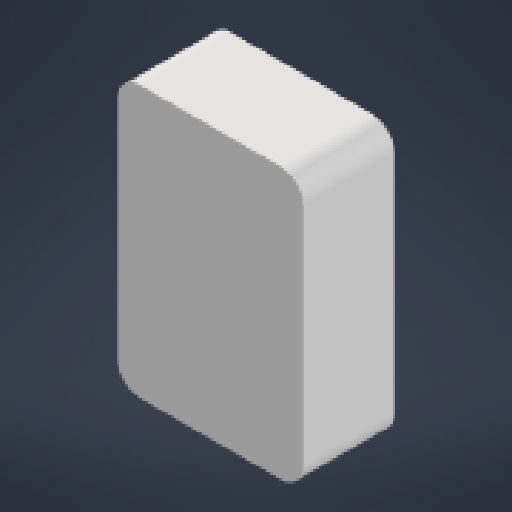
# Autodesk Inventor part: RPI
Saved by Autodesk Inventor 2026.1 (Build 301233020, 233B)
## iProperties
Created: 2025-10-22
Part Number: RPI
Material: Generic
Document SubType Name: Modeling
Designer: Malthe Sennels
Density: 1 g/cm^3
Appearance: Default
Author: Malthe Sennels
Autodesk Inventor part; units mm, degrees
ref_plane "YZ Plane" through (0, 0, 0) normal (1, 0, 0) x (0, 1, 0)
ref_plane "XZ Plane" through (0, 0, 0) normal (0, 1, 0) x (-1, 0, 0)
ref_plane "XY Plane" through (0, 0, 0) normal (0, 0, 1) x (1, 0, 0)
sketch "Sketch1" plane through (0, 0, 0) normal (0, 0, 1) x (1, 0, 0)
  line L0 (8, 0) -> (57, 0)
  line L1 (65, 8) -> (65, 87)
  line L2 (57, 95) -> (8, 95)
  line L3 (0, 87) -> (0, 8)
  arc A0 (0, 8) -> (8, 0) centre (8, 8) ccw
  arc A1 (8, 95) -> (0, 87) centre (8, 87) ccw
  arc A2 (65, 87) -> (57, 95) centre (57, 87) ccw
  arc A3 (57, 0) -> (65, 8) centre (57, 8) ccw
  point P0 (0, 0)
  point P1 (65, 95)
  point P2 (65, 0)
  point P3 (0, 95)
  dimension "d0" = 65
  dimension "d1" = 95
  dimension "d2" = 8
  constraints: 8 end point, 8 point on circle, 8 point on line, 8 tangent, 4 centre point, 3 equal radius, 2 parallel, 1 horizontal, 1 perpendicular
  measures "d0" distance of point (0, 95) point (65, 95)
  measures "d1" distance of point (65, 95) point (65, 0)
  measures "d2" radius of A0
extrude "Extrusion1" add sketch "Sketch1" along normal blind 32
sketch "Sketch2" plane through (0, 0, 0) normal (0, 0, -1) x (-1, 0, 0)
  line L0 (-8, 12) -> (-57, 12) construction
  line L1 (-57, 12) -> (-57, 70) construction
  line L2 (-57, 70) -> (-8, 70) construction
  line L3 (-8, 70) -> (-8, 12) construction
  line L4 (-8, 0) -> (-57, 0) projected
  line L5 (-32.5, 0) -> (-32.5, 94.8442) construction
  circle A0 centre (-57, 12) radius 1.5
  circle A1 centre (-57, 70) radius 1.5
  circle A2 centre (-8, 70) radius 1.5
  circle A3 centre (-8, 12) radius 1.5
  line L6 (-16.9436, 109.56) -> (-16.9436, 104.8114) projected
  line L7 (-40.3748, 104.8114) -> (-28.4573, 104.8114) projected
  line L8 (0.0184, 88.6231) -> (0.0184, 5.8494) projected
  line L9 (-28.0001, -10.2773) -> (-40.3748, -10.2773) projected
  line L10 (-16.9436, -10.2773) -> (-16.9436, -14.3057) projected
  line L11 (-21.9436, -19.3057) -> (-23.0001, -19.3057) projected
  line L12 (-28.0001, -14.3057) -> (-28.0001, -10.2773) projected
  line L13 (-40.3748, -10.2773) -> (-40.3748, -14.3057) projected
  line L14 (-45.3748, -19.3057) -> (-47.2671, -19.3057) projected
  line L15 (-52.2671, -14.3057) -> (-52.2671, -10.2773) projected
  line L16 (-64.9916, 6.3782) -> (-64.9916, 88.5882) projected
  line L17 (-52.2671, 104.8114) -> (-52.2671, 109.56) projected
  line L18 (-47.2671, 114.56) -> (-45.3748, 114.56) projected
  line L19 (-40.3748, 109.56) -> (-40.3748, 104.8114) projected
  line L20 (-28.4573, 104.8114) -> (-28.4573, 109.56) projected
  line L21 (-23.4573, 114.56) -> (-21.9436, 114.56) projected
  line L22 (-15.7324, 83.4806) -> (-23.5066, 91.204) projected
  arc A4 (-23.5066, 91.204) -> (-27.0305, 92.6569) centre (-27.0305, 87.6569) ccw projected
  line L23 (-27.0305, 92.6569) -> (-42.3584, 92.6569) projected
  arc A5 (-42.3584, 92.6569) -> (-45.8878, 91.1985) centre (-42.3584, 87.6569) ccw projected
  line L24 (-45.8878, 91.1985) -> (-50.0687, 87.0321) projected
  arc A6 (-50.0687, 87.0321) -> (-51.5393, 83.4904) centre (-46.5393, 83.4904) ccw projected
  line L25 (-51.5393, 83.4904) -> (-51.5393, 49.6697) projected
  arc A7 (-51.5393, 49.6697) -> (-49.6635, 45.7659) centre (-46.5393, 49.6697) ccw projected
  line L26 (-49.6635, 45.7659) -> (-44.7373, 41.8235) projected
  arc A8 (-44.7373, 41.8235) -> (-41.6131, 40.7274) centre (-41.6131, 45.7274) ccw projected
  line L27 (-41.6131, 40.7274) -> (-23.3988, 40.7274) projected
  arc A9 (-23.3988, 40.7274) -> (-20.0405, 42.0231) centre (-23.3988, 45.7274) ccw projected
  line L28 (-20.0405, 42.0231) -> (-15.898, 45.7787) projected
  arc A10 (-15.898, 45.7787) -> (-14.2563, 49.483) centre (-19.2563, 49.483) ccw projected
  line L29 (-14.2563, 49.483) -> (-14.2563, 79.9335) projected
  arc A11 (-14.2563, 79.9335) -> (-15.7324, 83.4806) centre (-19.2563, 79.9335) ccw projected
  line L30 (-14.2563, 9.4113) -> (-14.2563, 25.1215) projected
  arc A12 (-14.2563, 25.1215) -> (-16.1322, 29.0254) centre (-19.2563, 25.1215) ccw projected
  line L31 (-16.1322, 29.0254) -> (-19.9618, 32.0901) projected
  arc A13 (-19.9618, 32.0901) -> (-23.0859, 33.1863) centre (-23.0859, 28.1863) ccw projected
  line L32 (-23.0859, 33.1863) -> (-41.6879, 33.1863) projected
  arc A14 (-41.6879, 33.1863) -> (-44.5033, 32.3183) centre (-41.6879, 28.1863) ccw projected
  line L33 (-44.5033, 32.3183) -> (-49.3548, 29.0127) projected
  arc A15 (-49.3548, 29.0127) -> (-51.5393, 24.8807) centre (-46.5393, 24.8807) ccw projected
  line L34 (-51.5393, 24.8807) -> (-51.5393, 7.149) projected
  arc A16 (-51.5393, 7.149) -> (-50.9681, 4.8281) centre (-46.5393, 7.149) ccw projected
  line L35 (-50.9681, 4.8281) -> (-49.1556, 1.3694) projected
  arc A17 (-49.1556, 1.3694) -> (-44.7268, -1.3097) centre (-44.7268, 3.6903) ccw projected
  line L36 (-44.7268, -1.3097) -> (-23.7592, -1.3097) projected
  arc A18 (-23.7592, -1.3097) -> (-19.8301, 0.5979) centre (-23.7592, 3.6903) ccw projected
  line L37 (-19.8301, 0.5979) -> (-15.3273, 6.3189) projected
  arc A19 (-15.3273, 6.3189) -> (-14.2563, 9.4113) centre (-19.2563, 9.4113) ccw projected
  arc A20 (-64.9916, 6.3782) -> (-63.7832, 3.1188) centre (-59.9916, 6.3782) ccw projected
  arc A21 (-63.7296, 91.909) -> (-64.9916, 88.5882) centre (-59.9916, 88.5882) ccw projected
  line L38 (-63.7296, 91.909) -> (-52.2671, 104.8114) projected
  arc A22 (-47.2671, 114.56) -> (-52.2671, 109.56) centre (-47.2671, 109.56) ccw projected
  arc A23 (-40.3748, 109.56) -> (-45.3748, 114.56) centre (-45.3748, 109.56) ccw projected
  arc A24 (-23.4573, 114.56) -> (-28.4573, 109.56) centre (-23.4573, 109.56) ccw projected
  arc A25 (-16.9436, 109.56) -> (-21.9436, 114.56) centre (-21.9436, 109.56) ccw projected
  line L39 (-16.9436, 104.8114) -> (-1.8245, 92.5003) projected
  arc A26 (0.0184, 88.6231) -> (-1.8245, 92.5003) centre (-4.9816, 88.6231) ccw projected
  arc A27 (-1.834, 1.9645) -> (0.0184, 5.8494) centre (-4.9816, 5.8494) ccw projected
  line L40 (-1.834, 1.9645) -> (-16.9436, -10.2773) projected
  arc A28 (-21.9436, -19.3057) -> (-16.9436, -14.3057) centre (-21.9436, -14.3057) ccw projected
  arc A29 (-28.0001, -14.3057) -> (-23.0001, -19.3057) centre (-23.0001, -14.3057) ccw projected
  arc A30 (-45.3748, -19.3057) -> (-40.3748, -14.3057) centre (-45.3748, -14.3057) ccw projected
  arc A31 (-52.2671, -14.3057) -> (-47.2671, -19.3057) centre (-47.2671, -14.3057) ccw projected
  line L41 (-52.2671, -10.2773) -> (-63.7832, 3.1188) projected
  circle A32 centre (-57, 70) radius 2 projected
  circle A33 centre (-57, 12) radius 2 projected
  circle A34 centre (-8, 70) radius 2 projected
  circle A35 centre (-8, 12) radius 2 projected
  circle A36 centre (-22.639, 109.6569) radius 1.75 projected
  circle A37 centre (-46.639, -14.5983) radius 1.75 projected
  circle A38 centre (-46.639, 109.6569) radius 1.75 projected
  circle A39 centre (-22.639, -14.5983) radius 1.75 projected
  point P0 (0, 0)
  dimension "d5" = 49
  dimension "d6" = 58
  dimension "d7" = 24.5
  dimension "d8" = 12
  dimension "d9" = 3
  dimension "d10" = 3
  dimension "d11" = 3
  dimension "d12" = 3
  constraints: 10 end point, 4 centre point, 4 coincident, 2 parallel, 1 horizontal, 1 midpoint, 1 perpendicular, 1 vertical
  measures "d5" distance of L0.start L0.end
  measures "d6" distance between parallel lines of L0 L2
  measures "d7" distance between parallel lines of L1 L5
  measures "d8" distance between parallel lines of L4 L0
  measures "d9" diameter of A0
  measures "d10" diameter of A1
  measures "d11" diameter of A2
  measures "d12" diameter of A3
extrude "Extrusion2" cut sketch "Sketch2" against normal blind 10 contours A0 | A1 | A2 | A3
body "Solid1"
